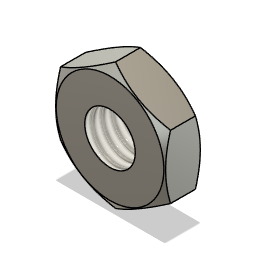
motor_module_v3 v19 (Autodesk Fusion 360 archive; units mm, degrees)
design "Hexagon Nut JIS B 1181 - M3 - Class 3 Finished Steel 6 Plain"
description: Hexagon Nut JIS B 1181 - M3 - Class 3 Finished
Autodesk Fusion 360 part; units mm, degrees
sketch "Sketch1" plane through (0, 0, 0) normal (0, 1, 0) x (1, 0, 0)
  line L0 (0, 0) -> (0, -1.8)
  line L1 (-1.5, 0) -> (-2.695, 0)
  line L2 (-2.695, 0) -> (-3.1763, -0.2778)
  line L3 (-3.1763, -0.2778) -> (-3.1763, -1.5222)
  line L4 (-3.1763, -1.5222) -> (-2.695, -1.8)
  line L5 (-2.695, -1.8) -> (-1.5, -1.8)
  line L6 (-1.5, -1.8) -> (-1.5, 0)
  dimension "d121" = 3
  dimension "d122" = 30
  dimension "d123" = 30
  dimension "d125" = 5.39
  dimension "d126" = 1.8
  dimension "d128" = 6.3525
  constraint vertical L0
  constraint coincident L0 L0.end
  constraint coincident origin L0
  constraint horizontal L1
  constraint perpendicular L1 L3
  constraint perpendicular L3 L5
  constraint perpendicular L5 L6
  constraint coincident L0.start L1
  constraint coincident L0.start origin
  constraint vertical L1.end L4.end
  constraint coincident L0.end L5
  measures "d122" angle of L1 L2
  measures "d123" angle of L4 L5
  measures "d126" distance of L1.start L5.end
revolve "Revolve1" add sketch "Sketch1" angle 360 about axis through (0, 0, 0) along (0, 0, 1)
sketch "Sketch8" plane through (0, 0, 1.8) normal (0, 0, 1) x (1, 0, 0)
  line L0 (0, 0) -> (-5.5, 0) construction
  line L1 (-2.75, -1.5894) -> (-2.75, 1.5894)
  circle A0 centre (0, 0) radius 1.5
  circle A1 centre (0, 0) radius 3.1763
  dimension "d114" = 2.75
  constraint horizontal L0
  constraint perpendicular L0 L1
  constraint midpoint L0 L1
  constraint coincident L0.start A0.centre
  constraint coincident L1.end A1
  measures "d114" distance of L0.start L1
extrude "Extrude5" cut sketch "Sketch8" against normal blind 1.8 contours L1 A1 picked at (-2.8188, -0.3871)
pattern_circular "C-Pattern2" count 6 over 360 about axis through (0, 0, 1.75) along (0, 0, 1) of "Extrude5"
thread "Thread3" "ISO Metric profile 3.0 M3x0.5 6H" major diameter 3.086 minor diameter 2.529 pitch 0.5 angle 60 resizes the face on face at (-1.4981, 0.0748, 1.2)
equation "adsk_nheig = 1.80 mm"
equation "adsk_maxdia = 6.3525 mm"
equation "adsk_nomdia = 3.00 mm"
equation "d89 = -adsk_nheig"
equation "adsk_waflat = 5.50 mm"
equation "d114 = adsk_waflat / 2"
equation "adsk_chamang1 = 30.00 deg"
equation "adsk_chamang2 = 30.00 deg"
equation "d121 = adsk_nomdia"
equation "d122 = adsk_chamang1"
equation "d123 = adsk_chamang2"
equation "d125 = adsk_beardia"
equation "d126 = adsk_nheig"
equation "d128 = adsk_maxdia"
equation "d147 = adsk_nheig"
equation "adsk_beardia = adsk_waflat * 0.98"

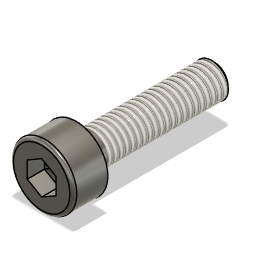
design "Broached Hexagon Socket Head Cap Screw ASME B18.3.1M - M3x0.5 x 12 Steel Grade 2 Plain"
description: Broached Hexagon Socket Head Cap Screw ASME B18.3.1M - M3x0.5 x 12
Autodesk Fusion 360 part; units mm, degrees
sketch "Sketch1" plane through (0, 0, 0) normal (0, 1, 0) x (1, 0, 0)
  line L0 (-1.5, 0) -> (-1.5, 12)
  line L1 (-1.5, 12) -> (0, 12)
  line L2 (0, 12) -> (0, -3)
  line L3 (-1.5, 0) -> (-2.75, 0)
  line L4 (-2.75, 0) -> (-2.75, -3)
  line L5 (-2.75, -3) -> (0, -3)
  dimension "d9" = 3
  dimension "d66" = 5.5
  dimension "d68" = 12
  dimension "d79" = 3
  constraint perpendicular L0 L1
  constraint collinear origin L1.end L2.end
  constraint perpendicular L0 L3
  constraint coincident origin L3
  constraint vertical L0
  constraint vertical L2
  constraint parallel L2 L4
  constraint coincident L2 L5.end
  constraint perpendicular L2 L5
  measures "d68" distance of origin L1.end
  measures "d79" distance of L3.end L4.end
revolve "Revolve1" add sketch "Sketch1" angle 360 about axis through (0, 0, -12) along (0, 0, 1)
ref_plane "WorkPlane1" through (0, 0, 3) normal (0, 0, 1) x (1, 0, 0)
sketch "Sketch6" plane through (0, 0, 3) normal (0, 0, 1) x (1, 0, 0)
  line L0 (-1.25, 0) -> (1.25, 0) construction
  line L1 (0, 0) -> (-1.25, 0.7217)
  line L2 (-1.25, -0.7217) -> (-1.25, 0.7217)
  line L3 (-1.25, -0.7217) -> (0, 0)
  dimension "d72" = 2.5
  dimension "d100" = 150
  constraint horizontal L0
  constraint midpoint L1.start L0
  constraint coincident L1.start L3.end
  constraint perpendicular L0 L2
  constraint midpoint L0.start L2
  constraint coincident L1.end L2.end
  measures "d72" distance of L0.start L0.end
  measures "d100" angle of L0 L1
extrude "Extrude1" cut sketch "Sketch6" against normal blind 1.5
pattern_circular "C-Pattern1" count 6 over 360 about axis through (0, 0, 1.75) along (0, 0, 1) of "Extrude1"
extrude "Extrude2" cut 1 faces at (0.4167, -0.2406, 1.5) along direction (0, 0, -1) blind 1.5 draft -85
thread "Thread2" "ANSI Metric M Profile 3.0 M3x0.5 4g6g" major diameter 2.927 minor diameter 2.369 pitch 0.5 angle 60 resizes the face on face at (-1.4981, 0.0748, -4) from (0, 0, -1.3067) to (0, 0, -12)
fillet "Fillet4" radius 0.3 1 edges at (-2.5639, 0.9944, 3)
sketch "Sketch7" plane through (0, 0, 0) normal (0, 1, 0) x (1, 0, 0)
  line L0 (-1.53, 12) -> (-1.53, 11.6933)
  line L1 (-1.53, 11.6933) -> (-1.1933, 12)
  line L2 (0, 12) -> (0, -3)
  line L3 (-1.53, 12) -> (0, 12)
  dimension "d92" = 0.3067
  dimension "d98" = 1.1933
  dimension "d99" = 1.53
  constraint coincident L2.start L3.end
  constraint perpendicular L2 L3
  constraint coincident L1.end L3
  constraint perpendicular L0 L3
  measures "d92" vertical distance of L0.end L1.end
  measures "d98" horizontal distance of origin L1.end
  measures "d99" distance of origin L0
revolve "Revolve3" cut sketch "Sketch7" angle 360 about axis through (0, 0, 1.75) along (0, 0, 1)
equation "d9 = adsk_nomdia"
equation "adsk_nomlen = 12.00 mm"
equation "adsk_headh = 3.00 mm"
equation "adsk_headdia = 5.50 mm"
equation "adsk_nomdia = 3.00 mm"
equation "adsk_philwidth = 2.50 mm"
equation "d31 = -adsk_phildepth"
equation "adsk_phildepth = 1.50 mm"
equation "d66 = adsk_headdia"
equation "d68 = adsk_nomlen"
equation "d71 = adsk_headh"
equation "d72 = adsk_philwidth"
equation "d76 = -adsk_phildepth"
equation "d79 = adsk_headh"
equation "adsk_thrlen = 10.693275 mm"
equation "d84 = adsk_thrlen"
equation "d86 = adsk_nomdia * 0.1"
equation "d92 = adsk_startlen"
equation "adsk_startlen = 0.306725 mm"
equation "adsk_endpointdia = 2.38655 mm"
equation "d98 = adsk_endpointdia / 2"
equation "d99 = adsk_nomdia * 0.51"

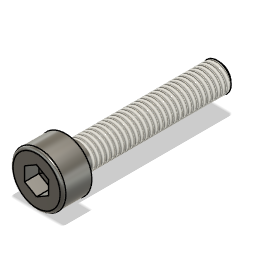
design "Broached Hexagon Socket Head Cap Screw ASME B18.3.1M - M3x0.5 x 16 Steel Grade 2 Plain"
description: Broached Hexagon Socket Head Cap Screw ASME B18.3.1M - M3x0.5 x 16
Autodesk Fusion 360 part; units mm, degrees
sketch "Sketch1" plane through (0, 0, 0) normal (0, 1, 0) x (1, 0, 0)
  line L0 (-1.5, 0) -> (-1.5, 16)
  line L1 (-1.5, 16) -> (0, 16)
  line L2 (0, 16) -> (0, -3)
  line L3 (-1.5, 0) -> (-2.75, 0)
  line L4 (-2.75, 0) -> (-2.75, -3)
  line L5 (-2.75, -3) -> (0, -3)
  dimension "d9" = 3
  dimension "d66" = 5.5
  dimension "d68" = 16
  dimension "d79" = 3
  constraint perpendicular L0 L1
  constraint collinear origin L1.end L2.end
  constraint perpendicular L0 L3
  constraint coincident origin L3
  constraint vertical L0
  constraint vertical L2
  constraint parallel L2 L4
  constraint coincident L2 L5.end
  constraint perpendicular L2 L5
  measures "d68" distance of origin L1.end
  measures "d79" distance of L3.end L4.end
revolve "Revolve1" add sketch "Sketch1" angle 360 about axis through (0, 0, -16) along (0, 0, 1)
ref_plane "WorkPlane1" through (0, 0, 3) normal (0, 0, 1) x (1, 0, 0)
sketch "Sketch6" plane through (0, 0, 3) normal (0, 0, 1) x (1, 0, 0)
  line L0 (-1.25, 0) -> (1.25, 0) construction
  line L1 (0, 0) -> (-1.25, 0.7217)
  line L2 (-1.25, -0.7217) -> (-1.25, 0.7217)
  line L3 (-1.25, -0.7217) -> (0, 0)
  dimension "d72" = 2.5
  dimension "d100" = 150
  constraint horizontal L0
  constraint midpoint L1.start L0
  constraint coincident L1.start L3.end
  constraint perpendicular L0 L2
  constraint midpoint L0.start L2
  constraint coincident L1.end L2.end
  measures "d72" distance of L0.start L0.end
  measures "d100" angle of L0 L1
extrude "Extrude1" cut sketch "Sketch6" against normal blind 1.5
pattern_circular "C-Pattern1" count 6 over 360 about axis through (0, 0, 1.75) along (0, 0, 1) of "Extrude1"
extrude "Extrude2" cut 1 faces at (0, -0.4811, 1.5) along direction (0, 0, -1) blind 1.5 draft -85
thread "Thread2" "ANSI Metric M Profile 3.0 M3x0.5 4g6g" major diameter 2.927 minor diameter 2.369 pitch 0.5 angle 60 resizes the face on face at (-1.4981, 0.0748, -5.3333) from (0, 0, -1.3067) to (0, 0, -16)
fillet "Fillet4" radius 0.3 1 edges at (-2.5639, 0.9944, 3)
sketch "Sketch7" plane through (0, 0, 0) normal (0, 1, 0) x (1, 0, 0)
  line L0 (-1.53, 16) -> (-1.53, 15.6933)
  line L1 (-1.53, 15.6933) -> (-1.1933, 16)
  line L2 (0, 16) -> (0, -3)
  line L3 (-1.53, 16) -> (0, 16)
  dimension "d92" = 0.3067
  dimension "d98" = 1.1933
  dimension "d99" = 1.53
  constraint coincident L2.start L3.end
  constraint perpendicular L2 L3
  constraint coincident L1.end L3
  constraint perpendicular L0 L3
  measures "d92" vertical distance of L0.end L1.end
  measures "d98" horizontal distance of origin L1.end
  measures "d99" distance of origin L0
revolve "Revolve3" cut sketch "Sketch7" angle 360 about axis through (0, 0, 1.75) along (0, 0, 1)
equation "d9 = adsk_nomdia"
equation "adsk_nomlen = 16.00 mm"
equation "adsk_headh = 3.00 mm"
equation "adsk_headdia = 5.50 mm"
equation "adsk_nomdia = 3.00 mm"
equation "adsk_philwidth = 2.50 mm"
equation "d31 = -adsk_phildepth"
equation "adsk_phildepth = 1.50 mm"
equation "d66 = adsk_headdia"
equation "d68 = adsk_nomlen"
equation "d71 = adsk_headh"
equation "d72 = adsk_philwidth"
equation "d76 = -adsk_phildepth"
equation "d79 = adsk_headh"
equation "adsk_thrlen = 14.693275 mm"
equation "d84 = adsk_thrlen"
equation "d86 = adsk_nomdia * 0.1"
equation "d92 = adsk_startlen"
equation "adsk_startlen = 0.306725 mm"
equation "adsk_endpointdia = 2.38655 mm"
equation "d98 = adsk_endpointdia / 2"
equation "d99 = adsk_nomdia * 0.51"

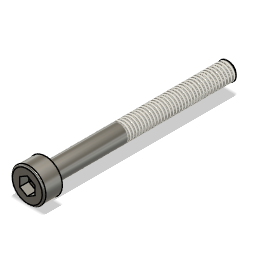
design "Broached Hexagon Socket Head Cap Screw ASME B18.3.1M - M3x0.5 x 30 Steel Grade 2 Plain"
description: Broached Hexagon Socket Head Cap Screw ASME B18.3.1M - M3x0.5 x 30
Autodesk Fusion 360 part; units mm, degrees
sketch "Sketch1" plane through (0, 0, 0) normal (0, 1, 0) x (1, 0, 0)
  line L0 (-1.5, 0) -> (-1.5, 30)
  line L1 (-1.5, 30) -> (0, 30)
  line L2 (0, 30) -> (0, -3)
  line L3 (-1.5, 0) -> (-2.75, 0)
  line L4 (-2.75, 0) -> (-2.75, -3)
  line L5 (-2.75, -3) -> (0, -3)
  dimension "d9" = 3
  dimension "d66" = 5.5
  dimension "d68" = 30
  dimension "d79" = 3
  constraint perpendicular L0 L1
  constraint collinear origin L1.end L2.end
  constraint perpendicular L0 L3
  constraint coincident origin L3
  constraint vertical L0
  constraint vertical L2
  constraint parallel L2 L4
  constraint coincident L2 L5.end
  constraint perpendicular L2 L5
  measures "d68" distance of origin L1.end
  measures "d79" distance of L3.end L4.end
revolve "Revolve1" add sketch "Sketch1" angle 360 about axis through (0, 0, -30) along (0, 0, 1)
ref_plane "WorkPlane1" through (0, 0, 3) normal (0, 0, 1) x (1, 0, 0)
sketch "Sketch6" plane through (0, 0, 3) normal (0, 0, 1) x (1, 0, 0)
  line L0 (-1.25, 0) -> (1.25, 0) construction
  line L1 (0, 0) -> (-1.25, 0.7217)
  line L2 (-1.25, -0.7217) -> (-1.25, 0.7217)
  line L3 (-1.25, -0.7217) -> (0, 0)
  dimension "d72" = 2.5
  dimension "d100" = 150
  constraint horizontal L0
  constraint midpoint L1.start L0
  constraint coincident L1.start L3.end
  constraint perpendicular L0 L2
  constraint midpoint L0.start L2
  constraint coincident L1.end L2.end
  measures "d72" distance of L0.start L0.end
  measures "d100" angle of L0 L1
extrude "Extrude1" cut sketch "Sketch6" against normal blind 1.5
pattern_circular "C-Pattern1" count 6 over 360 about axis through (0, 0, 1.75) along (0, 0, 1) of "Extrude1"
extrude "Extrude2" cut 1 faces at (0, -0.4811, 1.5) along direction (0, 0, -1) blind 1.5 draft -85
thread "Thread2" "ANSI Metric M Profile 3.0 M3x0.5 4g6g" major diameter 2.927 minor diameter 2.369 pitch 0.5 angle 60 resizes the face on face at (-1.4981, 0.0748, -10) from (0, 0, -12) to (0, 0, -30)
fillet "Fillet4" radius 0.3 1 edges at (-2.5639, 0.9944, 3)
sketch "Sketch7" plane through (0, 0, 0) normal (0, 1, 0) x (1, 0, 0)
  line L0 (-1.53, 30) -> (-1.53, 29.6933)
  line L1 (-1.53, 29.6933) -> (-1.1933, 30)
  line L2 (0, 30) -> (0, -3)
  line L3 (-1.53, 30) -> (0, 30)
  dimension "d92" = 0.3067
  dimension "d98" = 1.1933
  dimension "d99" = 1.53
  constraint coincident L2.start L3.end
  constraint perpendicular L2 L3
  constraint coincident L1.end L3
  constraint perpendicular L0 L3
  measures "d92" vertical distance of L0.end L1.end
  measures "d98" horizontal distance of origin L1.end
  measures "d99" distance of origin L0
revolve "Revolve3" cut sketch "Sketch7" angle 360 about axis through (0, 0, 1.75) along (0, 0, 1)
equation "d9 = adsk_nomdia"
equation "adsk_nomlen = 30.00 mm"
equation "adsk_headh = 3.00 mm"
equation "adsk_headdia = 5.50 mm"
equation "adsk_nomdia = 3.00 mm"
equation "adsk_philwidth = 2.50 mm"
equation "d31 = -adsk_phildepth"
equation "adsk_phildepth = 1.50 mm"
equation "d66 = adsk_headdia"
equation "d68 = adsk_nomlen"
equation "d71 = adsk_headh"
equation "d72 = adsk_philwidth"
equation "d76 = -adsk_phildepth"
equation "d79 = adsk_headh"
equation "adsk_thrlen = 18.00 mm"
equation "d84 = adsk_thrlen"
equation "d86 = adsk_nomdia * 0.1"
equation "d92 = adsk_startlen"
equation "adsk_startlen = 0.306725 mm"
equation "adsk_endpointdia = 2.38655 mm"
equation "d98 = adsk_endpointdia / 2"
equation "d99 = adsk_nomdia * 0.51"
